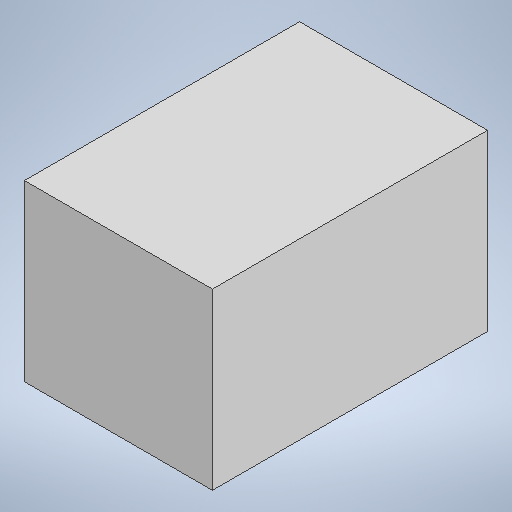
# Autodesk Inventor part: Part4
Saved by Autodesk Inventor 2026.2 (Build 302298010, 298A)
## iProperties
Created: 2026-05-20
Part Number: Part4
Material: 一般
Document SubType Name: Modeling
Designer: Yagis
Density: 1 g/cm^3
Appearance: 既定
Author: Yagis
Autodesk Inventor part; units mm, degrees
ref_plane "YZ Plane" through (0, 0, 0) normal (1, 0, 0) x (0, 1, 0)
ref_plane "XZ Plane" through (0, 0, 0) normal (0, 1, 0) x (-1, 0, 0)
ref_plane "XY Plane" through (0, 0, 0) normal (0, 0, 1) x (1, 0, 0)
sketch "スケッチ1" plane through (0, 0, 0) normal (1, 0, 0) x (0, 1, 0)
  line L0 (0, 0) -> (38, 0)
  line L1 (38, 0) -> (38, -60)
  line L2 (38, -60) -> (0, -60)
  line L3 (0, -60) -> (0, 0)
  dimension "d0" = 60
  dimension "d1" = 38
  constraints: 8 end point, 2 parallel, 1 horizontal, 1 perpendicular
  measures "d0" distance of L2.end L0.start
  measures "d1" distance of L1.end L2.end
extrude "押し出し1" add sketch "スケッチ1" along normal blind 41
sketch "スケッチ4" plane through (0, 0, 0) normal (-1, 0, 0) x (0, 0, 1)
  line L0 (0, 0) -> (-60, 0) projected
  line L1 (0, 38) -> (0, 0) projected
  point P0 (-29, 34)
  point P1 (-9, 34)
  point P2 (-9, 4)
  point P3 (-29, 4)
  dimension "d4" = 20
  dimension "d5" = 30
  dimension "d7" = 9
  dimension "d15" = 4
  constraints: 2 horizontal alignment, 2 vertical alignment
  measures "d4" distance of point (-29, 4) point (-9, 4)
  measures "d5" distance of point (-9, 4) point (-9, 34)
  measures "d7" distance from line of L1 point (-9, 4)
  measures "d15" distance from line of L0 point (-9, 4)
hole "穴1" at (0, 34, -29) at (0, 34, -9) at (0, 4, -9) at (0, 4, -29) direction (1, 0, 0) diameter 2.459 depth 8.8 tip angle 118 thread size "M3x0.5" class "6H" standard "ISO Metric profile"
